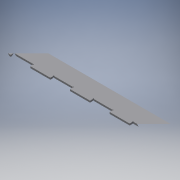
# Autodesk Inventor part: frente inferior
Saved by Autodesk Inventor 2016 (Build 200138000, 138)
## iProperties
Created: 2017-06-07
Part Number: frente inferior
Material: Generic
Document SubType Name: Modeling
Designer: fabio-note
Density: 1 g/cm^3
Appearance: Default
Author: fabio-note
Autodesk Inventor part; units mm, degrees
ref_plane "YZ Plane" through (0, 0, 0) normal (1, 0, 0) x (0, 1, 0)
ref_plane "XZ Plane" through (0, 0, 0) normal (0, 1, 0) x (-1, 0, 0)
ref_plane "XY Plane" through (0, 0, 0) normal (0, 0, 1) x (1, 0, 0)
sketch "Sketch1" plane through (0, 0, 0) normal (0, 0, 1) x (1, 0, 0)
  line L0 (-173, 24) -> (173, 24)
  line L1 (173, 24) -> (173, -24)
  line L2 (173, -24) -> (-173, -24)
  line L3 (-173, -24) -> (-173, 24)
  point P0 (0, 0)
  point P1 (173, 0)
  point P2 (0, 24)
  dimension "d0" = 48
  dimension "d1" = 346
  constraints: 8 end point, 2 midpoint, 2 parallel, 1 horizontal, 1 horizontal alignment, 1 perpendicular, 1 vertical alignment
  measures "d0" distance between parallel lines of L2 L0
  measures "d1" distance between parallel lines of L3 L1
extrude "Extrusion1" add sketch "Sketch1" along normal blind 4
sketch "Esboço2" plane through (0, 0, 4) normal (0, 0, 1) x (1, 0, 0)
  line L0 (-165, -24) -> (-118.5, -24)
  line L1 (-118.5, -24) -> (-118.5, -16)
  line L2 (-118.5, -16) -> (-165, -16)
  line L3 (-165, -16) -> (-165, -24)
  line L4 (-173, 24) -> (-173, -24) projected
  line L5 (-70.5, -24) -> (-24, -24)
  line L6 (-24, -24) -> (-24, -16)
  line L7 (-24, -16) -> (-70.5, -16)
  line L8 (-70.5, -16) -> (-70.5, -24)
  circle A0 centre (-24, -16) radius 1
  circle A1 centre (-70.5, -16) radius 1
  circle A2 centre (-118.5, -16) radius 1
  circle A3 centre (-165, -16) radius 1
  line L9 (-173, -24) -> (173, -24) projected
  point P0 (0, 0)
  dimension "d4" = 46.5
  dimension "d7" = 46.5
  dimension "d8" = 48
  dimension "d14" = 2
  dimension "d15" = 2
  dimension "d16" = 2
  dimension "d20" = 8
  dimension "d21" = 8
  dimension "d22" = 0
  constraints: 16 end point, 4 centre point, 4 coincident, 4 parallel, 2 horizontal, 2 perpendicular
  measures "d4" distance of L2.end L1.end
  measures "d7" distance of L7.end L6.end
  measures "d8" distance between parallel lines of L8 L1
  measures "d14" diameter of A0
  measures "d15" diameter of A1
  measures "d16" diameter of A2
  measures "d20" distance between parallel lines of L3 L4
  measures "d21" distance between parallel lines of L0 L2
  measures "d22" distance between parallel lines of L9 L0
extrude "Extrusão2" cut sketch "Esboço2" against normal blind 10
mirror "Espelhamento1" about plane through (0, 0, 0) normal (1, 0, 0) of "Extrusão2"
sketch "Esboço3" plane through (0, 0, 4) normal (0, 0, 1) x (1, 0, 0)
  line L0 (-173, 24) -> (-173, -24) projected
  line L1 (-173, -8) -> (-165, -8)
  line L2 (-165, -8) -> (-165, 8)
  line L3 (-165, 8) -> (-173, 8)
  line L4 (-173, 8) -> (-173, -8)
  line L5 (-173, -24) -> (-165, -24) projected
  line L6 (173, 24) -> (-173, 24) projected
  circle A0 centre (-165, 8) radius 1
  circle A1 centre (-165, -8) radius 1
  point P0 (0, 0)
  dimension "d23" = 8
  dimension "d24" = 16
  dimension "d25" = 16
  dimension "d26" = 16
  dimension "d27" = 2
  dimension "d28" = 2
  constraints: 8 end point, 2 centre point, 2 coincident, 2 parallel, 1 horizontal, 1 perpendicular, 1 point on line
  measures "d23" distance of L3.end L2.end
  measures "d24" distance between parallel lines of L3 L1
  measures "d25" distance between parallel lines of L5 L1
  measures "d26" distance between parallel lines of L6 L3
  measures "d27" diameter of A0
  measures "d28" diameter of A1
extrude "Extrusão3" cut sketch "Esboço3" against normal blind 10
mirror "Espelhamento2" about plane through (0, 0, 0) normal (1, 0, 0) of "Extrusão3"
body "Solid1"
